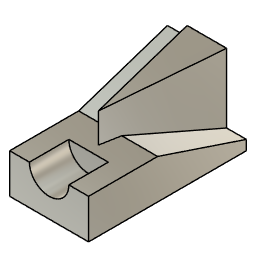
32 (Autodesk Fusion 360 design; units mm, degrees)
Autodesk Fusion 360 part; units mm, degrees
sketch "草图1" plane through (0, 0, 0) normal (0, 0, 1) x (1, 0, 0)
  line L0 (-100, 87.5) -> (100, 87.5)
  line L1 (100, 87.5) -> (100, -87.5)
  line L2 (100, -87.5) -> (-100, -87.5)
  line L3 (-100, -87.5) -> (-100, 87.5)
  line L4 (-100, 0) -> (100, 0) construction
  line L5 (0, 75) -> (0, -50) construction
  dimension "d1" = 200
  dimension "d2" = 175
  constraint horizontal L0
  constraint vertical L1
  constraint horizontal L2
  constraint vertical L3
  constraint horizontal L4
  constraint vertical L5
  constraint symmetric L0 L2 L4
  constraint symmetric L1 L3 L5
  measures "d1" distance of L0.start L0.end
  measures "d2" distance of L0.end L1.end
extrude "拉伸1" add sketch "草图1" against normal blind 100
sketch "草图2" plane through (0, -87.5, 0) normal (0, -1, 0) x (1, 0, 0)
  line L0 (100, 0) -> (-100, 0)
  line L1 (-100, 0) -> (-100, -100)
  line L2 (-100, -100) -> (100, -100)
  line L3 (100, -100) -> (100, 0)
  circle A0 centre (0, 0) radius 50
  dimension "d5" = 100
  constraint coincident A0.centre origin
  measures "d5" diameter of A0
extrude "拉伸2" cut sketch "草图2" against normal blind 100 contours L0 A0 picked at (10.3915, -13.0305)
sketch "草图3" plane through (100, 0, 0) normal (1, 0, 0) x (0, 1, 0)
  line L0 (87.5, 0) -> (-87.5, 0)
  line L1 (-87.5, 0) -> (-87.5, -100)
  line L2 (-87.5, -100) -> (87.5, -100)
  line L3 (87.5, -100) -> (87.5, 0)
  line L4 (87.5, 0) -> (312.5, -75)
  line L5 (312.5, -75) -> (312.5, -100)
  line L6 (312.5, -100) -> (87.5, -100)
  line L7 (-150, 0) -> (245.1978, 0) construction
  dimension "d8" = 25
  dimension "d9" = 225
  constraint coincident L0.start L3.end
  constraint perpendicular L0 L5
  constraint coincident L2.end L3.start
  constraint perpendicular L1 L7
  constraint parallel L6 L7
  measures "d8" distance of L4.end L5.end
  measures "d9" distance of L5.end L2.end
extrude "拉伸3" add sketch "草图3" against normal blind 100 contours L3 L4 L5 L6
sketch "草图4" plane through (-100, 0, 0) normal (-1, 0, 0) x (0, -1, 0)
  line L0 (87.5, 0) -> (-87.5, 0)
  line L1 (-87.5, 0) -> (-87.5, -100)
  line L2 (-87.5, -100) -> (87.5, -100)
  line L3 (87.5, -100) -> (87.5, 0)
  line L4 (-312.5, 75) -> (-87.5, 0)
  line L5 (-87.5, -100) -> (-312.5, -100)
  line L6 (-312.5, -100) -> (-312.5, 75)
  dimension "d12" = 175
  dimension "d13" = 225
  constraint coincident L0.end L1.start
  constraint coincident L1.end L2.start
  constraint perpendicular L1 L5
  constraint perpendicular L5 L6
  measures "d12" distance of L4.start L5.end
  measures "d13" distance of L1.end L5.end
extrude "拉伸4" add sketch "草图4" against normal blind 100 contours L1 L4 L5 L6
ref_plane "工作平面1" through (0, 0, 100) normal (0, 0, 1) x (1, 0, 0)
sketch "草图5" plane through (0, 0, 100) normal (0, 0, 1) x (1, 0, 0)
  line L0 (-50, 312.5) -> (50, 312.5)
  line L1 (50, 312.5) -> (0, 37.5)
  line L2 (0, 37.5) -> (-50, 312.5)
  line L3 (0, -125) -> (0, 391.0284) construction
  point P0 (100, -87.5)
  point P1 (-100, -87.5)
  point P2 (-100, 87.5)
  point P3 (100, 87.5)
  point P4 (-100, 312.5)
  point P5 (100, 312.5)
  dimension "d17" = 275
  dimension "d18" = 100
  constraint horizontal L0
  constraint perpendicular L0 L3
  constraint collinear P4 P5 L0.start
  constraint collinear L1.end L3.start L3.end
  constraint symmetric L0.start L0.end L3
  measures "d17" distance of L0 L1.end
  measures "d18" distance of L0.start L0.end
extrude "拉伸5" add sketch "草图5" against normal through all
sketch "草图6" plane through (100, 0, 0) normal (1, 0, 0) x (0, 1, 0)
  line L0 (87.5, 0) -> (-87.5, 0)
  line L1 (-87.5, 0) -> (-87.5, -100)
  line L2 (-87.5, -100) -> (312.5, -100)
  line L3 (312.5, -100) -> (312.5, -75)
  line L4 (312.5, -75) -> (87.5, 0)
  line L5 (37.5, 100) -> (37.5, 93.4578)
  line L6 (37.5, 93.4578) -> (37.5, 75)
  line L7 (37.5, 75) -> (312.5, 100)
  line L8 (312.5, 100) -> (37.5, 100)
  point P0 (37.5, 100)
  point P1 (312.5, 100)
  dimension "d20" = 25
  constraint coincident P0 L5.start
  constraint vertical L5
  constraint parallel L5 L6
  constraint coincident P1 L7.end
  measures "d20" distance of P0 L6.end
extrude "拉伸6" cut sketch "草图6" against normal blind 375 contours L5 L6 L7 L8
equation "d2 = 400 mm - 225 mm"
